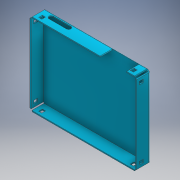
# Autodesk Inventor part: metal_cover_connector
Saved by Autodesk Inventor 2018 (Build 220112000, 112)
## iProperties
Created: 2019-04-18
Part Number: metal_cover_connector
Material: Generic
Document SubType Name: Modeling
Designer: ZEUSLAP
Density: 1 g/cm^3
Appearance: Default
Author: ZEUSLAP
Autodesk Inventor part; units mm, degrees
ref_plane "YZ Plane" through (0, 0, 0) normal (1, 0, 0) x (0, 1, 0)
ref_plane "XZ Plane" through (0, 0, 0) normal (0, 1, 0) x (-1, 0, 0)
ref_plane "XY Plane" through (0, 0, 0) normal (0, 0, 1) x (1, 0, 0)
sketch "Sketch3" plane through (0, 0, 0) normal (0, 1, 0) x (-1, 0, 0)
  line L0 (23, 18.5) -> (-23, 18.5)
  line L1 (-24, 17.5) -> (-24, -17.5)
  line L2 (-23, -18.5) -> (23, -18.5)
  line L3 (24, -17.5) -> (24, 17.5)
  line L4 (24, 18.5) -> (-24, -18.5) construction
  circle A0 centre (24, 18.5) radius 1
  circle A1 centre (24, -18.5) radius 1
  circle A2 centre (-24, -18.5) radius 1
  circle A3 centre (-24, 18.5) radius 1
  point P0 (0, 0)
  dimension "d21" = 2
  dimension "d22" = 2
  dimension "d23" = 2
  dimension "d24" = 2
  constraints: 10 end point, 8 point on circle, 4 centre point, 2 coincident, 2 parallel, 1 horizontal, 1 midpoint, 1 perpendicular
  measures "d21" diameter of A0
  measures "d22" diameter of A1
  measures "d23" diameter of A2
  measures "d24" diameter of A3
extrude "Extrusion3" add sketch "Sketch3" along normal blind 0.5 contours A0 L3 A1 L2 A2 L1 A3 L0
sketch "Sketch6" plane through (0, 0, 0) normal (0, -1, 0) x (1, 0, 0)
  line L0 (-23, 18.5) -> (23, 18.5) projected
  line L1 (-23, 18.5) -> (23, 18.5)
  line L2 (24, 17.5) -> (24, -17.5) projected
  line L3 (24, 17.5) -> (24, -17.5)
  line L4 (-24, -17.5) -> (-24, 17.5) projected
  line L5 (-24, -17.5) -> (-24, 17.5)
  circle A0 centre (-24, 18.5) radius 1
  circle A1 centre (24, 18.5) radius 1
  circle A2 centre (24, -18.5) radius 1
  circle A3 centre (-24, -18.5) radius 1
  line L6 (23.5, -17.634) -> (23.5, 17.634)
  line L7 (-23.134, 18) -> (23.134, 18)
  line L8 (-23.5, -17.634) -> (-23.5, 17.634)
  line L9 (23, -18.5) -> (-23, -18.5) projected
  line L10 (-23, -18.5) -> (23, -18.5)
  line L11 (23.134, -18) -> (-23.134, -18)
  point P0 (0, 0)
  dimension "d45" = 0.5
  dimension "d46" = 0.5
  dimension "d48" = 2
  dimension "d49" = 0.5
  constraints: 16 end point, 14 point on circle, 4 centre point, 4 collinear, 3 parallel, 1 point on line
  measures "d45" distance between parallel lines of L0 L7
  measures "d46" distance between parallel lines of L4 L8
  measures "d48" diameter of A3
  measures "d49" distance between parallel lines of L9 L11
extrude "Extrusion5" add sketch "Sketch6" along normal blind 5.5 contours L0 A1 L7 A0 | A0 L8 A3 L4 | L2 A2 L6 A1 | A3 L11 A2 L9
sketch "Sketch7" plane through (-23, 0.5, 18.5) normal (0, 0, 1) x (1, 0, 0)
  line L0 (42.9, -3.1) -> (44.3, -3.1)
  line L1 (44.3, -3.1) -> (44.3, -4.8)
  line L2 (44.3, -4.8) -> (42.9, -4.8)
  line L3 (42.9, -4.8) -> (42.9, -3.1)
  line L4 (0, 0) -> (46, 0) projected
  line L5 (46, -6) -> (46, 0) projected
  line L6 (1.7, -3.1) -> (3.1, -3.1)
  line L7 (3.1, -3.1) -> (3.1, -4.8)
  line L8 (3.1, -4.8) -> (1.7, -4.8)
  line L9 (1.7, -4.8) -> (1.7, -3.1)
  line L10 (0, 0) -> (0, -6) projected
  point P0 (23, -0.5)
  dimension "d52" = 1.4
  dimension "d53" = 1.7
  dimension "d54" = 3.1
  dimension "d55" = 1.7
  dimension "d56" = 1.4
  dimension "d57" = 1.7
  dimension "d58" = 3.1
  dimension "d59" = 1.7
  constraints: 16 end point, 4 parallel, 2 horizontal, 2 perpendicular
  measures "d52" distance of L1.end L2.end
  measures "d53" distance of L0.end L1.end
  measures "d54" distance between parallel lines of L0 L4
  measures "d55" distance between parallel lines of L1 L5
  measures "d56" distance of L7.end L8.end
  measures "d57" distance of L6.end L7.end
  measures "d58" distance between parallel lines of L6 L4
  measures "d59" distance between parallel lines of L10 L9
extrude "Extrusion6" cut sketch "Sketch7" against normal up to surface (37 mm away)
sketch "Sketch8" plane through (24, 0.5, 17.5) normal (1, 0, 0) x (0, 0, -1)
  line L0 (32.4, -3.1) -> (33.8, -3.1)
  line L1 (33.8, -3.1) -> (33.8, -4.8)
  line L2 (33.8, -4.8) -> (32.4, -4.8)
  line L3 (32.4, -4.8) -> (32.4, -3.1)
  line L4 (0, 0) -> (35, 0) projected
  line L5 (35, -6) -> (35, 0) projected
  line L6 (1.2, -3.1) -> (2.6, -3.1)
  line L7 (2.6, -3.1) -> (2.6, -4.8)
  line L8 (2.6, -4.8) -> (1.2, -4.8)
  line L9 (1.2, -4.8) -> (1.2, -3.1)
  line L10 (0, -6) -> (0, 0) projected
  point P0 (17.5, -0.5)
  dimension "d62" = 1.4
  dimension "d63" = 1.7
  dimension "d64" = 3.1
  dimension "d65" = 1.2
  dimension "d66" = 1.4
  dimension "d67" = 1.7
  dimension "d68" = 3.1
  dimension "d69" = 1.2
  constraints: 16 end point, 4 parallel, 2 horizontal, 2 perpendicular
  measures "d62" distance of L1.end L2.end
  measures "d63" distance of L0.end L1.end
  measures "d64" distance between parallel lines of L4 L0
  measures "d65" distance between parallel lines of L5 L1
  measures "d66" distance of L7.end L8.end
  measures "d67" distance of L6.end L7.end
  measures "d68" distance between parallel lines of L4 L6
  measures "d69" distance between parallel lines of L10 L9
extrude "Extrusion7" cut sketch "Sketch8" against normal up to surface (48 mm away)
sketch "Sketch10" plane through (-23, 0.5, 18.5) normal (0, 0, 1) x (1, 0, 0)
  line L0 (42.5, -0.5) -> (30.5, -0.5)
  line L1 (30.5, -0.5) -> (30.5, -6)
  line L2 (30.5, -6) -> (42.5, -6)
  line L3 (42.5, -6) -> (42.5, -0.5)
  line L4 (0, 0) -> (46, 0) projected
  line L5 (46, -6) -> (46, 0) projected
  line L6 (4.5, -1) -> (12.4, -1)
  line L7 (13.4, -2) -> (13.4, -2)
  line L8 (12.4, -3) -> (4.5, -3)
  line L9 (3.5, -2) -> (3.5, -2)
  line L10 (0, 0) -> (0, -6) projected
  arc A0 (13.4, -2) -> (12.4, -1) centre (12.4, -2) ccw
  arc A1 (12.4, -3) -> (13.4, -2) centre (12.4, -2) ccw
  arc A2 (3.5, -2) -> (4.5, -3) centre (4.5, -2) ccw
  arc A3 (4.5, -1) -> (3.5, -2) centre (4.5, -2) ccw
  line L11 (46, -6) -> (0, -6) projected
  point P0 (23, -0.5)
  point P1 (13.4, -3)
  point P2 (13.4, -1)
  point P3 (3.5, -3)
  dimension "d80" = 12
  dimension "d81" = 5.5
  dimension "d82" = 0.5
  dimension "d83" = 3.5
  dimension "d84" = 9.9
  dimension "d85" = 2
  dimension "d87" = 3.5
  dimension "d88" = 1
  dimension "d89" = 1
  dimension "d90" = 1
  dimension "d94" = 3
  constraints: 16 end point, 8 point on circle, 8 tangent, 6 point on line, 4 centre point, 4 parallel, 2 horizontal, 2 perpendicular, 1 concentric
  measures "d80" distance of L2.end L1.end
  measures "d81" distance of L1.end L0.end
  measures "d82" distance between parallel lines of L0 L4
  measures "d83" distance between parallel lines of L3 L5
  measures "d84" distance of point (13.4, -3) point (3.5, -3)
  measures "d85" distance of point (13.4, -1) point (13.4, -3)
  measures "d87" distance between parallel lines of L9 L10
  measures "d88" radius of A0
  measures "d89" radius of A1
  measures "d90" radius of A2
  measures "d94" distance between parallel lines of L11 L8
extrude "Extrusion9" cut sketch "Sketch10" against normal up to surface (0.5 mm away) contours L3 L2 L1 L0 | L6 A0 A1 L8 A2 A3
fillet "Fillet1" radius 0.5 4 edges at (0, 0.5, 18.5) (-24, 0.5, 0) (24, 0.5, 0) (0, 0.5, -18.5)
body "Solid3"
